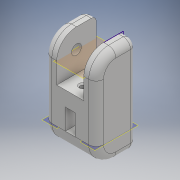
# Autodesk Inventor part: Falange-Distal
Saved by Autodesk Inventor 2018 (Build 220112000, 112)
## iProperties
Created: 2017-06-03
Part Number: Falange-Distal
Material: Genérico
Document SubType Name: Modeling
Designer: Vitor
Density: 1 g/cm^3
Appearance: Padrão
Author: Vitor
Autodesk Inventor part; units mm, degrees
ref_plane "YZ Plane" through (0, 0, 0) normal (1, 0, 0) x (0, 1, 0)
ref_plane "XZ Plane" through (0, 0, 0) normal (0, 1, 0) x (-1, 0, 0)
ref_plane "XY Plane" through (0, 0, 0) normal (0, 0, 1) x (1, 0, 0)
sketch "Esboço14" plane through (0, 0, 0) normal (0, 0, 1) x (1, 0, 0)
  line L0 (0, 0) -> (21, 0)
  line L1 (21, 0) -> (21, -16)
  line L2 (21, -16) -> (0, -16)
  line L3 (0, -16) -> (0, 0)
  dimension "d47" = 21
  dimension "d48" = 16
  constraints: 8 end point, 2 parallel, 1 horizontal, 1 perpendicular
  measures "d47" distance of L1.end L2.end
  measures "d48" distance of L0.end L1.end
extrude "Extrusão14" add sketch "Esboço14" along normal blind 6
sketch "Esboço15" plane through (21, -16, 0) normal (1, 0, 0) x (0, 0, -1)
  line L0 (-6, 0) -> (-14.5, 0)
  line L1 (-14.5, 0) -> (-14.5, 16)
  line L2 (-14.5, 16) -> (-6, 16)
  line L3 (-6, 16) -> (-6, 0)
  circle A0 centre (-14.5, 8) radius 8
  point P0 (0, 16)
  dimension "d123" = 8.5
  dimension "d124" = 16
  constraints: 8 end point, 2 parallel, 1 horizontal, 1 midpoint, 1 perpendicular, 1 vertical alignment, 2 other
  measures "d123" distance of L1.end L2.end
  measures "d124" distance of L0.end L1.end
extrude "Extrusão15" add sketch "Esboço15" against normal blind 5
sketch "Esboço16" plane through (0, -16, 0) normal (-1, 0, 0) x (0, 0, 1)
  line L0 (6, 16) -> (6, 0) projected
  line L1 (6, 16) -> (14.5, 16)
  line L2 (14.5, 16) -> (14.5, 0)
  line L3 (14.5, 0) -> (6, 0)
  line L4 (6, 0) -> (6, 16)
  circle A0 centre (14.5, 8) radius 8
  point P0 (15, 16)
  point P1 (15, 0)
  point P2 (15, 8)
  dimension "d121" = 8.5
  dimension "d122" = 16
  constraints: 8 end point, 2 parallel, 1 horizontal, 1 midpoint, 1 perpendicular, 1 vertical alignment, 2 other
  measures "d121" distance of L2.end L3.end
  measures "d122" distance of L1.end L2.end
extrude "Extrusão16" add sketch "Esboço16" against normal blind 5
sketch "Esboço17" plane through (0, 0, 0) normal (0, 0, -1) x (-1, 0, 0)
  line L0 (-16, 0) -> (-5, 0) projected
  line L1 (-10.5, 0) -> (-10.5, -16)
  line L2 (-21, -16) -> (0, -16) projected
  line L3 (-10.5, -16) -> (-8.5, -16)
  line L4 (-8.5, -16) -> (-8.5, 0)
  line L5 (-8.5, 0) -> (-12.5, 0)
  line L6 (-12.5, 0) -> (-12.5, -16)
  line L7 (-15.5, -8) -> (-15.5, -6)
  line L8 (-15.5, -8) -> (-13.5, -8) construction
  line L9 (-15.5, -6) -> (-8.5, -6)
  line L10 (-8.5, -6) -> (-5.5, -6)
  line L11 (-5.5, -6) -> (-5.5, -10)
  line L12 (-5.5, -10) -> (-15.5, -10)
  line L13 (-15.5, -10) -> (-15.5, -8)
  line L14 (-15.5, -6) -> (-12.5, -6)
  line L15 (-12.5, -10) -> (-12.5, -6)
  line L16 (-8.5, -6) -> (-8.5, -10)
  point P0 (0, 0)
  dimension "d57" = 2
  dimension "d58" = 4
  dimension "d60" = 2
  dimension "d61" = 90
  dimension "d62" = 3
  dimension "d63" = 4
  constraints: 30 end point, 10 point on line, 9 perpendicular, 2 midpoint, 1 collinear, 1 horizontal, 1 vertical
  measures "d57" distance of L1.end L3.end
  measures "d58" distance of L4.end L5.end
  measures "d60" distance of L7.start L7.end
  measures "d61" angle of L8 L7
  measures "d62" distance of L9.end L10.end
  measures "d63" distance of L10.end L11.end
extrude "Extrusão17" add sketch "Esboço17" along normal blind 8.5 contours L9 L1 L12 L6 | L6 L12 L13 L7 L9 | L9 L4 L12 L1 | L10 L11 L12 L4
sketch "Esboço18" plane through (5.5, -10, 0) normal (-1, 0, 0) x (0, 0, 1)
  line L0 (-8.5, 0) -> (-8.5, 4) projected
  circle A0 centre (-8.5, 2) radius 8
  line L1 (-8.5, 10) -> (0, 10)
  line L2 (0, -6) -> (0, 10) projected
  line L3 (0, 10) -> (0, -6)
  line L4 (0, -6) -> (-8.5, -6)
  dimension "d66" = 16
  constraints: 6 end point, 2 point on circle, 1 centre point, 1 midpoint, 1 perpendicular, 1 tangent
  measures "d66" diameter of A0
extrude "Extrusão18" add sketch "Esboço18" against normal blind 3
sketch "Esboço19" plane through (15.5, -10, 0) normal (1, 0, 0) x (0, 0, -1)
  line L0 (8.5, 4) -> (8.5, 0) projected
  circle A0 centre (8.5, 2) radius 8
  line L1 (0, 10) -> (8.5, 10) projected
  line L2 (8.5, 10) -> (0, 10)
  line L3 (0, 10) -> (0, -6) projected
  line L4 (0, 10) -> (0, -6)
  line L5 (8.5, -6) -> (0, -6) projected
  line L6 (0, -6) -> (8.5, -6)
  constraints: 6 end point, 3 collinear, 1 centre point, 1 midpoint, 1 point on circle, 1 point on line
extrude "Extrusão19" add sketch "Esboço19" against normal blind 3
sketch "Esboço20" plane through (0, 0, 0) normal (0, 0, -1) x (-1, 0, 0)
  line L0 (-8.5, -10) -> (-12.5, -10) projected
  line L1 (-10.5, -10) -> (-10.5, -11)
  line L2 (-8.5, -6) -> (-12.5, -6) projected
  line L3 (-10.5, -6) -> (-10.5, -5)
  circle A0 centre (-10.5, -5) radius 1
  circle A1 centre (-10.5, -11) radius 1
  point P0 (0, 0)
  dimension "d72" = 1
  dimension "d73" = 1
  dimension "d74" = 2
  dimension "d75" = 2
  constraints: 4 end point, 2 centre point, 2 coincident, 2 midpoint, 2 vertical
  measures "d72" distance of L1.start L1.end
  measures "d73" distance of L3.start L3.end
  measures "d74" diameter of A0
  measures "d75" diameter of A1
extrude "Extrusão20" cut sketch "Esboço20" against normal blind 8
chamfer "Chanfro1" distance 0.5 angle 45 2 edges at (11.5, -5, 6) (11.5, -11, 6)
fillet "Arredondamento7" radius 0.5 4 edges at (9.7929, -5.7071, 0) (11.2071, -4.2929, 0) (9.7929, -10.2929, 0) (11.2071, -11.7071, 0)
ref_plane "Plano de trabalho1" through (0, 0, -8.5) normal (0, 0, -1) x (-1, 0, 0)
sketch "Esboço21" plane through (0, 0, -8.5) normal (0, 0, -1) x (-1, 0, 0)
  line L0 (-15.5, -16) -> (-15.5, 0) projected
  line L1 (-15.5, -8) -> (-16.5, -8)
  line L2 (-15.5, -8) -> (-15.5, -10)
  arc A0 (-16.5, -8) -> (-15.5, -10) centre (-14.5168, -8.2584) ccw
  point P0 (0, 0)
  dimension "d83" = 1
  dimension "d84" = 2
  dimension "d85" = 2
  constraints: 4 end point, 2 point on circle, 1 centre point, 1 horizontal, 1 midpoint, 1 point on line
  measures "d83" distance of L1.start L1.end
  measures "d84" distance of L1.start L2.end
  measures "d85" radius of A0
revolve "Revolução1" add sketch "Esboço21" angle 360 about axis through (15.5, -8, -8.5) along (1, 0, 0)
ref_plane "Plano de trabalho2" through (0, 0, -8.5) normal (0, 0, -1) x (-1, 0, 0)
ref_plane "Plano de trabalho3" through (0, 0, 14.5) normal (0, 0, 1) x (1, 0, 0)
sketch "Esboço23" plane through (0, 0, 14.5) normal (0, 0, 1) x (1, 0, 0)
  line L0 (16, -16) -> (16, 0) projected
  line L1 (16, -8) -> (17, -8)
  line L2 (16, -8) -> (16, -10)
  line L3 (5, 0) -> (5, -16) projected
  line L4 (5, -8) -> (4, -8)
  line L5 (5, -8) -> (5, -6)
  arc A0 (5, -6) -> (4, -8) centre (5.9832, -7.7416) ccw
  arc A1 (16, -10) -> (17, -8) centre (15.0168, -8.2584) ccw
  point P0 (0, 0)
  dimension "d93" = 1
  dimension "d94" = 2
  dimension "d95" = 1
  dimension "d96" = 2
  dimension "d97" = 2
  dimension "d98" = 2
  constraints: 8 end point, 4 point on circle, 2 centre point, 2 horizontal, 2 midpoint, 2 point on line
  measures "d93" distance of L1.start L1.end
  measures "d94" distance of L1.start L2.end
  measures "d95" distance of L4.start L4.end
  measures "d96" distance of L4.start L5.end
  measures "d97" radius of A0
  measures "d98" radius of A1
revolve "Revolução3" cut sketch "Esboço23" angle 360 about axis through (16, -8, 14.5) along (1, 0, 0)
sketch "Esboço28" plane through (21, -16, 0) normal (1, 0, 0) x (0, 0, -1)
  arc A0 (-14.5, 16) -> (-14.5, 0) centre (-14.5, 8) ccw projected
  line L0 (-14.5, 8) -> (-22.5, 8)
  line L1 (-22.5, 8) -> (-22.5, 16)
  line L2 (-22.5, 16) -> (-14.5, 16)
  line L3 (-14.5, 16) -> (-14.5, 8)
  line L4 (-14.5, 16) -> (-22.5, 8)
  point P0 (0, 16)
  dimension "d125" = 8
  dimension "d126" = 8
  constraints: 10 end point, 2 parallel, 1 horizontal, 1 perpendicular
  measures "d125" distance of L1.end L2.end
  measures "d126" distance of L0.end L1.end
extrude "Extrusão25" add sketch "Esboço28" against normal blind 5 contours L4 A0 | A0 L1 L2
sketch "Esboço29" plane through (0, -16, 0) normal (-1, 0, 0) x (0, 0, 1)
  arc A0 (14.5, 0) -> (22.5, 8) centre (14.5, 8) ccw projected
  line L0 (22.5, 8) -> (22.5, 16) projected
  line L1 (14.5, 8) -> (22.5, 8)
  line L2 (22.5, 8) -> (22.5, 16)
  line L3 (22.5, 16) -> (14.5, 16)
  line L4 (14.5, 16) -> (14.5, 8)
  line L5 (22.5, 8) -> (14.5, 16)
  point P0 (0, 16)
  constraints: 10 end point, 2 parallel, 1 horizontal, 1 perpendicular
extrude "Extrusão26" add sketch "Esboço29" against normal blind 5 contours L5 L3 L0
sketch "Esboço30" plane through (0, 0, -8.5) normal (0, 0, -1) x (-1, 0, 0)
  line L0 (-5.5, 0) -> (-5.5, -16) projected
  line L1 (-5.5, -8) -> (-4.5, -8)
  line L2 (-5.5, -8) -> (-5.5, -6)
  arc A0 (-4.5, -8) -> (-5.5, -6) centre (-6.4832, -7.7416) ccw
  point P0 (0, 0)
  dimension "d131" = 1
  dimension "d132" = 2
  dimension "d133" = 2
  constraints: 4 end point, 2 point on circle, 1 centre point, 1 horizontal, 1 midpoint, 1 point on line
  measures "d131" distance of L1.start L1.end
  measures "d132" distance of L1.start L2.end
  measures "d133" radius of A0
revolve "Revolução4" add sketch "Esboço30" angle 360 about axis through (5.5, -8, -8.5) along (-1, 0, 0)
sketch "Esboço31" plane through (15.5, -16, 0) normal (1, 0, 0) x (0, 0, -1)
  arc A0 (8.5, 0) -> (8.5, 16) centre (8.5, 8) ccw projected
  line L0 (16.5, 8) -> (16.5, 16)
  line L1 (16.5, 16) -> (8.5, 16)
  line L2 (0, 16) -> (8.5, 16) projected
  line L3 (16.5, 8) -> (8.5, 16)
  constraints: 6 end point
extrude "Extrusão27" add sketch "Esboço31" against normal blind 3
sketch "Esboço32" plane through (5.5, -16, 0) normal (-1, 0, 0) x (0, 0, 1)
  arc A0 (-16.5, 8) -> (-8.5, 0) centre (-8.5, 8) ccw projected
  line L0 (-8.5, 8) -> (-16.5, 8)
  line L1 (-16.5, 8) -> (-16.5, 16)
  line L2 (-16.5, 16) -> (-8.5, 16)
  line L3 (-8.5, 16) -> (-8.5, 8)
  line L4 (0, 16) -> (-8.5, 16) projected
  line L5 (-8.5, 16) -> (-16.5, 8)
  constraints: 10 end point, 2 parallel, 1 horizontal, 1 perpendicular
extrude "Extrusão28" add sketch "Esboço32" against normal blind 3 contours L1 L2 L5
sketch "Esboço33" plane through (0, 0, 6) normal (0, 0, 1) x (1, 0, 0)
  line L0 (5, 0) -> (5, -16) projected
  line L1 (16, -16) -> (16, 0) projected
  line L2 (5, 0) -> (16, 0)
  line L3 (10.5, 0) -> (10.5, -1.6)
  circle A0 centre (10.5, -1.6) radius 1.5
  point P0 (0, 0)
  dimension "d141" = 1.6
  dimension "d142" = 3
  constraints: 4 end point, 1 centre point, 1 coincident, 1 horizontal, 1 midpoint, 1 vertical
  measures "d141" distance of L3.start L3.end
  measures "d142" diameter of A0
extrude "Extrusão29" add sketch "Esboço33" along normal blind 4
fillet "Arredondamento8" radius 1.5 1 edges at (9, -1.6, 10)
sketch "Esboço34" plane through (0, 0, 0) normal (0, 0, -1) x (-1, 0, 0)
  circle A0 centre (-10.5, -1.6) radius 1.5 projected
  circle A1 centre (-10.5, -1.6) radius 1.5
  point P0 (0, 0)
  dimension "d146" = 3
  constraints: 1 centre point, 1 coincident
  measures "d146" diameter of A1
extrude "Extrusão30" add sketch "Esboço34" along normal blind 4
fillet "Arredondamento9" radius 1.5 1 edges at (12, -1.6, -4)
sketch "Esboço35" plane through (0, 0, 0) normal (0, 0, -1) x (-1, 0, 0)
  line L0 (-16, 0) -> (-5, 0) projected
  arc A0 (-9.7682, -2.9094) -> (-11.2318, -2.9094) centre (-10.5, 0) ccw
  circle A1 centre (-10.5, -1.6) radius 1.5 projected
  circle A2 centre (-10.5, -1.6) radius 1.5
  circle A3 centre (-10.5, -1.6) radius 1.5 projected
  circle A4 centre (-10.5, -1.6) radius 1.5
  point P0 (0, 0)
  dimension "d150" = 6
  constraints: 4 point on circle, 3 centre point, 2 coincident, 1 midpoint
  measures "d150" diameter of A0
extrude "Extrusão31" cut sketch "Esboço35" along normal blind 4 contours A0 L0 | L0 A0 A1
fillet "Arredondamento10" radius 0.5 8 edges at (13, 0, -4) (12.5, -1.118, -4) (12.5, 0, -10.25) (8.5, 0, -10.25) (8, 0, -4) (8.5, -1.118, -4) (8.5, -2.2361, -2) (12.5, -2.2361, -2)
sketch "Esboço36" plane through (5.5, -16, 0) normal (-1, 0, 0) x (0, 0, 1)
  line L0 (0, 16) -> (-16.5, 16) projected
  arc A0 (-16.5, 8) -> (-8.5, 0) centre (-8.5, 8) ccw projected
  line L1 (0, 16) -> (-16.5, 16)
  line L2 (-16.5, 16) -> (-16.5, 8)
  line L3 (-16.5, 8) -> (0, 8)
  line L4 (0, 8) -> (0, 16)
  line L5 (0, 16) -> (0, 0) projected
  line L6 (-8.5, 8) -> (0, 8)
  line L7 (0, 8) -> (0, 0)
  line L8 (0, 0) -> (-8.5, 0)
  line L9 (-8.5, 0) -> (-8.5, 8)
  circle A1 centre (-8.5, 8) radius 8
  constraints: 16 end point, 4 parallel, 2 horizontal, 2 perpendicular, 1 coincident, 1 horizontal alignment, 2 other
extrude "Extrusão32" add sketch "Esboço36" along normal blind 5.5
sketch "Esboço37" plane through (15.5, -16, 0) normal (1, 0, 0) x (0, 0, -1)
  line L0 (16.5, 16) -> (-22.5, 16) projected
  line L1 (0, 0) -> (8.5, 0) projected
  line L2 (16.5, 16) -> (0, 16)
  line L3 (0, 16) -> (0, 0)
  line L4 (0, 0) -> (8.5, 0)
  line L5 (16.5, 8) -> (16.5, 16)
  circle A0 centre (8.5, 8) radius 2 projected
  arc A1 (8.5, 0) -> (16.5, 8) centre (8.5, 8) ccw projected
  circle A2 centre (8.5, 8) radius 8
  constraints: 8 end point, 3 point on circle, 2 parallel, 1 centre point, 1 coincident, 1 horizontal, 1 perpendicular
extrude "Extrusão33" add sketch "Esboço37" along normal blind 5.5 contours L5 A2 L0 | A2 L1 L3 L0 | A2 A1 | A0
sketch "Esboço38" plane through (8.5, -10, 0) normal (1, 0, 0) x (0, 0, -1)
  line L0 (4.5, 10) -> (16.5, 10) projected
  arc A0 (6.5, 0) -> (6.5, 4) centre (6.5, 2) ccw projected
  line L1 (16.5, 10) -> (8.5, 10)
  line L2 (8.5, 10) -> (8.5, 2)
  line L3 (8.5, 2) -> (16.5, 2)
  line L4 (16.5, 2) -> (16.5, 10)
  arc A1 (8.5, -6) -> (16.5, 2) centre (8.5, 2) ccw projected
  circle A2 centre (8.5, 2) radius 8
  line L5 (8.5, -6) -> (8.5, 2)
  line L6 (8.5, 2) -> (16.5, 2)
  point P0 (0, 10)
  constraints: 12 end point, 3 equal length, 1 coincident, 1 horizontal, 1 perpendicular, 1 point on circle, 1 tangent, 1 vertical, 1 vertical alignment, 2 other
extrude "Extrusão34" add sketch "Esboço38" along normal blind 5.5 and the other way blind 2.75 contours A2 L3 L2 | L0 L4 A2 | L3 A1 L5
fillet "Arredondamento11" radius 3 12 edges at (0, -4, -16.5) (0, -13.6569, -14.1569) (0, -16, 7.25) (0, -16, -4.25) (0, -13.6569, 20.1569) (0, -4, 22.5) (21, -13.6569, -14.1569) (21, -16, -4.25) (21, -16, 7.25) (21, -13.6569, 20.1569) (21, -4, 22.5) (21, -4, -16.5)
fillet "Arredondamento12" radius 2 17 edges at (20.1213, 0, -15.6213) (21, 0, -6.75) (21, 0, 9.75) (20.1213, 0, 21.6213) (17, 0, 22.5) (0.8787, 0, -15.6213) (0, 0, 9.75) (0, 0, -6.75) (0.8787, 0, 21.6213) (4, 0, 22.5) (16.75, 0, -16.5) (14.75, 0, -16.5) (13.5, 0, -16.5) (10.5, 0, -16.5) (6.875, 0, -16.5) (5.625, 0, -16.5) (4.25, 0, -16.5)
sketch "Esboço39" plane through (0, 0, 6) normal (0, 0, 1) x (1, 0, 0)
  arc A0 (13, 0) -> (12.5, -0.5) centre (13, -0.5) ccw projected
  line L0 (7.9184, -3.2281) -> (13, -3.2281)
  line L1 (13, -3.2281) -> (13, 0)
  line L2 (13, 0) -> (7.9184, 0)
  line L3 (7.9184, 0) -> (7.9184, -3.2281)
  point P0 (0, 0)
  constraints: 8 end point, 2 parallel, 1 horizontal, 1 perpendicular, 1 point on circle
extrude "Extrusão35" cut sketch "Esboço39" along normal blind 10
sketch "Esboço40" plane through (0, 0, 6) normal (0, 0, 1) x (1, 0, 0)
  arc A0 (11.618, -6) -> (9.382, -6) centre (10.5, -5) ccw projected
  circle A1 centre (10.5, -5) radius 1.5
  point P0 (0, 0)
  constraints: 1 centre point, 1 coincident
extrude "Extrusão36" add sketch "Esboço40" against normal blind 6
sketch "Esboço41" plane through (16, -16, 0) normal (-1, 0, 0) x (0, 0, 1)
  line L0 (19.5, 16) -> (20.5, 16) projected
  line L1 (22.5, 14) -> (22.5, 8) projected
  line L2 (19.5, 16) -> (22.5, 16)
  line L3 (22.5, 16) -> (22.5, 8)
  line L4 (22.5, 8) -> (19.5, 8)
  line L5 (19.5, 8) -> (19.5, 16)
  point P0 (0, 16)
  constraints: 8 end point, 2 parallel, 1 horizontal, 1 perpendicular
